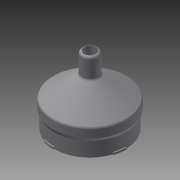
# Autodesk Inventor part: screwflare74
Saved by Autodesk Inventor 2014 SP1 (Build 180222100, 222)
## iProperties
Created: 2014-04-21
Part Number: screwflare74
Material: Generic
Document SubType Name: Modeling
Designer: lukeiseman
Density: 1 g/cm^3
Appearance: Default
Author: lukeiseman
Autodesk Inventor part; units mm, degrees
ref_plane "YZ Plane" through (0, 0, 0) normal (1, 0, 0) x (0, 1, 0)
ref_plane "XZ Plane" through (0, 0, 0) normal (0, 1, 0) x (-1, 0, 0)
ref_plane "XY Plane" through (0, 0, 0) normal (0, 0, 1) x (1, 0, 0)
sketch "Sketch2" plane through (0, 0, 0) normal (0, 0, 1) x (1, 0, 0)
  line L0 (0, 0) -> (0, 25.4)
  line L1 (0, 25.4) -> (7.62, 25.4)
  line L2 (7.62, 25.4) -> (9.144, 25.4)
  line L3 (10.9873, 24.8102) -> (46.2933, -0.3635)
  line L4 (40.6545, 1.846) -> (7.62, 25.4)
  line L5 (47.625, -2.9486) -> (47.625, -12.4656)
  line L6 (10.9873, 24.8102) -> (11.4917, 24.4504)
  line L7 (9.144, 25.4) -> (10.16, 25.4)
  line L8 (10.16, 27.0356) -> (10.16, 47.625)
  line L9 (7.62, 50.8) -> (7.62, 25.4)
  line L10 (45.9232, -2.5626) -> (45.9232, -11.4526)
  arc A0 (10.16, 47.625) -> (7.62, 50.7359) centre (6.985, 47.625) ccw
  arc A1 (47.625, -2.9486) -> (46.2933, -0.3635) centre (44.45, -2.9486) ccw
  arc A2 (10.16, 27.0356) -> (11.4917, 24.4504) centre (13.335, 27.0356) ccw
  line L11 (40.6545, 1.846) -> (45.9232, -2.5626)
  line L12 (47.625, -12.4656) -> (45.9232, -11.4526)
  line L13 (45.9232, -2.5626) -> (45.9232, -11.4526)
  line L14 (45.5168, -35.3256) -> (45.5168, -16.9106)
  line L15 (47.625, -12.4656) -> (52.4025, -12.4656) construction
  line L16 (43.8086, -35.3256) -> (43.8086, -15.9112)
  line L17 (45.9232, -2.5626) -> (45.9232, -11.4526)
  line L18 (45.5168, -35.3256) -> (43.8086, -35.3256)
  line L19 (45.5168, -16.9106) -> (45.5168, -35.3256)
  line L20 (47.625, -12.4656) -> (45.5168, -16.9106)
  line L21 (45.9232, -11.4526) -> (43.8086, -15.9112)
  line L22 (7.62, 25.4) -> (3.81, 25.4)
  line L23 (3.81, 25.4) -> (3.81, 32.3365)
  line L24 (7.62, 25.4) -> (3.81, 28.1166)
  line L25 (3.81, 28.1166) -> (7.62, 28.1166)
  point P0 (47.625, -1.313)
  point P1 (10.16, 50.8)
  point P2 (46.1518, -17.3808)
  point P3 (44.9154, -1.7193)
  point P4 (46.1518, -15.158)
  point P5 (42.6103, 0.2095)
  dimension "d9" = 25.4
  dimension "d10" = 7.62
  dimension "d11" = 2.54
  dimension "d16" = 25.4
  dimension "d18" = 3.175
  dimension "d19" = 3.175
  dimension "d24" = 47.625
  dimension "d26" = 8.89
  dimension "d53" = 45.5168
  dimension "d55" = 1.7082
  dimension "d56" = 22.86
  dimension "d68" = 1.7018
  dimension "d84" = 18.415
  dimension "d86" = 3.81
  constraints: 52 end point, 14 point on line, 7 point on circle, 6 perpendicular, 5 tangent, 4 parallel, 3 centre point, 3 collinear, 1 equal radius, 1 horizontal, 1 midpoint
  measures "d9" distance of L0.start L0.end
  measures "d10" distance of L0.end L1.end
  measures "d11" distance of L1.end L7.end
  measures "d16" distance of L7.end point (10.16, 50.8)
  measures "d18" radius of A0
  measures "d19" radius of A2
  measures "d24" distance between parallel lines of L0 L5
  measures "d26" distance of L10.end L10.start
  measures "d53" distance between parallel lines of L0 L14
  measures "d55" distance between parallel lines of L14 L16
  measures "d56" vertical distance of L14.start L5.end
  measures "d68" distance between parallel lines of L5 L10
  measures "d84" distance of L14.start L14.end
  measures "d86" distance of L1.end L22.end
ref_plane "Work Plane1" through (0, -36.5956, 0) normal (0, -1, 0) x (1, 0, 0)
revolve "Revolution5" add sketch "Sketch2" angle 360 about axis through (0, 0, 0) along (0, 1, 0) contours L9 A0 L8 A2 L3 A1 L5 L12 L10 L11 L4 | L24 L25 L9 | L12 L20 L14 L18 L16 L21
sketch "Sketch8" plane through (0, -35.3256, 0) normal (0, -1, 0) x (1, 0, 0)
  circle A0 centre (0, 0) radius 43.8086 projected
  line L0 (0, 43.8086) -> (0, 46.5836)
  line L1 (41.6644, 13.5376) -> (44.3484, 14.2568)
  line L2 (43.8086, 0) -> (46.5836, 0) construction
  line L3 (0, 0) -> (46.5836, 0)
  line L4 (-13.6758, 41.6193) -> (-14.3951, 44.3036)
  line L5 (0, 0) -> (46.5836, 0) construction
  line L6 (-43.8086, 0) -> (-46.5836, 0)
  line L7 (-41.6193, -13.6758) -> (-44.3036, -14.3951)
  line L8 (0, 0) -> (46.5836, 0) construction
  line L9 (0, -43.8086) -> (0, -46.5836)
  line L10 (13.5376, -41.6644) -> (14.2568, -44.3484)
  line L11 (0, 0) -> (46.5836, 0) construction
  arc A1 (0, 46.5836) -> (-14.3951, 44.3036) centre (0, 0) ccw
  arc A2 (-46.5836, 0) -> (-44.3036, -14.3951) centre (0, 0) ccw
  arc A3 (0, -46.5836) -> (14.2568, -44.3484) centre (0, 0) ccw
  arc A4 (46.5836, 0) -> (44.3484, 14.2568) centre (0, 0) ccw
  arc A5 (0, -43.8086) -> (13.5376, -41.6644) centre (0, 0) ccw
  arc A6 (-43.8086, 0) -> (-41.6193, -13.6758) centre (0, 0) ccw
  arc A7 (43.8086, 0) -> (41.6644, 13.5376) centre (0, 0) ccw
  arc A8 (0, 43.8086) -> (-13.6758, 41.6193) centre (0, 0) ccw
  line L12 (46.5836, 0) -> (43.8086, 0)
  circle A9 centre (0, 0) radius 45.5168 projected
  circle A10 centre (0, 0) radius 41.275
  dimension "d72" = 15
  dimension "d75" = 105
  dimension "d78" = 165
  dimension "d81" = 75
  dimension "d85" = 82.55
  constraints: 26 end point, 16 point on circle, 9 centre point, 9 coincident, 4 horizontal, 4 perpendicular, 3 collinear, 1 vertical, 9 other
  measures "d72" angle of L2 L1
  measures "d75" angle of L5 L4
  measures "d78" angle of L7 L8
  measures "d81" angle of L10 L11
  measures "d85" diameter of A10
extrude "Extrusion7" add sketch "Sketch8" against normal blind 2.54 contours A0 | A0 L1 A9 L3 | L10 A9 L9 A0 | A9 L1 A4 L3 | A0 L4 A9 L0 | L10 A3 L9 A9 | A9 L4 A1 L0 | L7 A9 L6 A0 | L7 A2 L6 A9
body "Solid3"
